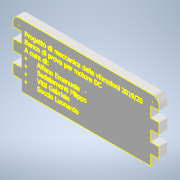
# Autodesk Inventor part: base
Saved by Autodesk Inventor 2020.2 (Build 242310000, 310)
## iProperties
Created: 2020-02-13
Part Number: base
Material: Generico
Document SubType Name: Modeling
Designer: socci
Density: 1 g/cm^3
Appearance: Default
Author: socci
Autodesk Inventor part; units mm, degrees
(part 1 of 5)
ref_plane "YZ Plane" through (0, 0, 0) normal (1, 0, 0) x (0, 1, 0)
ref_plane "XZ Plane" through (0, 0, 0) normal (0, 1, 0) x (-1, 0, 0)
ref_plane "XY Plane" through (0, 0, 0) normal (0, 0, 1) x (1, 0, 0)
sketch "Schizzo1" plane through (0, 0, 0) normal (0, 0, 1) x (1, 0, 0)
  line L0 (-35, -15) -> (35, -15)
  line L1 (35, -15) -> (35, 12)
  line L2 (32, 15) -> (-32, 15)
  line L3 (-35, 12) -> (-35, -15)
  line L4 (-35, -15) -> (35, 15) construction
  line L5 (35, -15) -> (-35, 15) construction
  arc A0 (-32, 15) -> (-35, 12) centre (-32, 12) ccw
  arc A1 (35, 12) -> (32, 15) centre (32, 12) ccw
  point P0 (0, 0)
  dimension "d0" = 70
  dimension "d1" = 30
  dimension "d6" = 3
  constraints: 12 end point, 4 point on circle, 4 point on line, 4 tangent, 2 centre point, 2 midpoint, 2 parallel, 1 equal radius, 1 horizontal, 1 perpendicular
  measures "d0" distance of L4.end L5.end
  measures "d1" distance of L5.end L0.start
  measures "d6" radius of A0
extrude "Estrusione1" add sketch "Schizzo1" along normal blind 4
sketch "Schizzo2" plane through (0, 0, 4) normal (0, 0, 1) x (1, 0, 0)
  line L0 (-29.4007, 10.8975) -> (27.8158, 10.8975) construction
  line L1 (27.8158, 10.8975) -> (27.8158, -22.4613) construction
  line L2 (27.8158, -22.4613) -> (-29.4007, -22.4613) construction
  line L3 (-29.4007, -22.4613) -> (-29.4007, 10.8975) construction
  line L4 (-31, -5) -> (-35, -5)
  line L5 (-35, -5) -> (-35, 0)
  line L6 (-35, 0) -> (-31, 0)
  line L7 (-31, 0) -> (-31, -5)
  line L8 (-35, 10) -> (-31, 10)
  line L9 (-31, 10) -> (-31, 5)
  line L10 (-31, 5) -> (-35, 5)
  line L11 (-35, 5) -> (-35, 10)
  line L12 (-31, -15) -> (-35, -15)
  line L13 (-35, -15) -> (-35, -10)
  line L14 (-35, -10) -> (-31, -10)
  line L15 (-31, -10) -> (-31, -15)
  line L16 (35, -5) -> (31, -5)
  line L17 (31, -5) -> (31, 0)
  line L18 (31, 0) -> (35, 0)
  line L19 (35, 0) -> (35, -5)
  line L20 (31, 10) -> (35, 10)
  line L21 (35, 10) -> (35, 5)
  line L22 (35, 5) -> (31, 5)
  line L23 (31, 5) -> (31, 10)
  line L24 (35, -15) -> (31, -15)
  line L25 (31, -15) -> (31, -10)
  line L26 (31, -10) -> (35, -10)
  line L27 (35, -10) -> (35, -15)
  arc A0 (35, 12) -> (32, 15) centre (32, 12) ccw
  line L28 (35, 12) -> (35, -15)
  line L29 (35, -15) -> (-35, -15)
  line L30 (-35, -15) -> (-35, 12)
  arc A1 (-32, 15) -> (-35, 12) centre (-32, 12) ccw
  line L31 (-32, 15) -> (32, 15)
  spline S0 degree 2 poles (-27.9339, 10.2055) (-27.9339, 10.0758) (-28.0263, 9.8424) (-28.109, 9.7614) knots 0 0 0 1 2 2 2
  spline S1 degree 2 poles (-28.109, 9.7614) (-28.2127, 9.6593) (-28.4931, 9.5539) (-28.707, 9.5539) knots 0 0 0 1 2 2 2
  line L32 (-28.707, 9.5539) -> (-28.9323, 9.5539)
  line L33 (-28.9323, 9.5539) -> (-28.9323, 8.8084)
  line L34 (-28.9323, 8.8084) -> (-29.1981, 8.8084)
  line L35 (-29.1981, 8.8084) -> (-29.1981, 10.8084)
  line L36 (-29.1981, 10.8084) -> (-28.6957, 10.8084)
  spline S2 degree 2 poles (-28.6957, 10.8084) (-28.5174, 10.8084) (-28.2678, 10.75) (-28.1722, 10.6836) knots 0 0 0 1 2 2 2
  spline S3 degree 2 poles (-28.1722, 10.6836) (-28.0603, 10.6074) (-27.9339, 10.3724) (-27.9339, 10.2055) knots 0 0 0 1 2 2 2
  spline S4 degree 2 poles (-28.2111, 10.1974) (-28.2111, 10.3011) (-28.2824, 10.4534) (-28.3553, 10.5021) knots 0 0 0 1 2 2 2
  spline S5 degree 2 poles (-28.3553, 10.5021) (-28.4185, 10.5442) (-28.5871, 10.5782) (-28.7119, 10.5782) knots 0 0 0 1 2 2 2
  line L37 (-28.7119, 10.5782) -> (-28.9323, 10.5782)
  line L38 (-28.9323, 10.5782) -> (-28.9323, 9.7808)
  line L39 (-28.9323, 9.7808) -> (-28.7508, 9.7808)
  spline S6 degree 2 poles (-28.7508, 9.7808) (-28.5887, 9.7808) (-28.3893, 9.8327) (-28.3245, 9.9008) knots 0 0 0 1 2 2 2
  spline S7 degree 2 poles (-28.3245, 9.9008) (-28.2646, 9.9607) (-28.2111, 10.1017) (-28.2111, 10.1974) knots 0 0 0 1 2 2 2
  line L40 (-26.9047, 10.0385) -> (-26.9177, 10.0385)
  spline S8 degree 2 poles (-26.9177, 10.0385) (-26.9469, 10.0466) (-27.0101, 10.0499) (-27.0539, 10.0499) knots 0 0 0 1 2 2 2
  spline S9 degree 2 poles (-27.0539, 10.0499) (-27.156, 10.0499) (-27.3569, 9.9607) (-27.4477, 9.8732) knots 0 0 0 1 2 2 2
  line L41 (-27.4477, 9.8732) -> (-27.4477, 8.8084)
  line L42 (-27.4477, 8.8084) -> (-27.7005, 8.8084)
  line L43 (-27.7005, 8.8084) -> (-27.7005, 10.3092)
  line L44 (-27.7005, 10.3092) -> (-27.4477, 10.3092)
  line L45 (-27.4477, 10.3092) -> (-27.4477, 10.0855)
  spline S10 degree 2 poles (-27.4477, 10.0855) (-27.3099, 10.2087) (-27.1041, 10.3092) (-27.0069, 10.3092) knots 0 0 0 1 2 2 2
  spline S11 degree 2 poles (-27.0069, 10.3092) (-26.968, 10.3092) (-26.9291, 10.306) (-26.9047, 10.3011) knots 0 0 0 1 2 2 2
  line L46 (-26.9047, 10.3011) -> (-26.9047, 10.0385)
  spline S12 degree 2 poles (-25.4752, 9.5588) (-25.4752, 9.1795) (-25.8399, 8.7662) (-26.1446, 8.7662) knots 0 0 0 1 2 2 2
  spline S13 degree 2 poles (-26.1446, 8.7662) (-26.4574, 8.7662) (-26.8156, 9.1925) (-26.8156, 9.5588) knots 0 0 0 1 2 2 2
  spline S14 degree 2 poles (-26.8156, 9.5588) (-26.8156, 9.9348) (-26.4461, 10.3513) (-26.1446, 10.3513) knots 0 0 0 1 2 2 2
  spline S15 degree 2 poles (-26.1446, 10.3513) (-25.8399, 10.3513) (-25.4752, 9.9364) (-25.4752, 9.5588) knots 0 0 0 1 2 2 2
  spline S16 degree 2 poles (-25.7362, 9.5588) (-25.7362, 9.8505) (-25.9485, 10.1342) (-26.1446, 10.1342) knots 0 0 0 1 2 2 2
  spline S17 degree 2 poles (-26.1446, 10.1342) (-26.3407, 10.1342) (-26.5547, 9.8505) (-26.5547, 9.5588) knots 0 0 0 1 2 2 2
  spline S18 degree 2 poles (-26.5547, 9.5588) (-26.5547, 9.2752) (-26.3407, 8.9834) (-26.1446, 8.9834) knots 0 0 0 1 2 2 2
  spline S19 degree 2 poles (-26.1446, 8.9834) (-25.9501, 8.9834) (-25.7362, 9.2703) (-25.7362, 9.5588) knots 0 0 0 1 2 2 2
  spline S20 degree 2 poles (-25.1624, 8.5685) (-25.1365, 8.5572) (-25.0376, 8.5215) (-24.9744, 8.5069) knots 0 0 0 1 2 2 2
  spline S21 degree 2 poles (-24.9744, 8.5069) (-24.9047, 8.4891) (-24.7864, 8.468) (-24.7167, 8.468) knots 0 0 0 1 2 2 2
  spline S22 degree 2 poles (-24.7167, 8.468) (-24.6, 8.468) (-24.438, 8.5296) (-24.3926, 8.5847) knots 0 0 0 1 2 2 2
  spline S23 degree 2 poles (-24.3926, 8.5847) (-24.3488, 8.6398) (-24.3148, 8.7841) (-24.3148, 8.8765) knots 0 0 0 1 2 2 2
  line L47 (-24.3148, 8.8765) -> (-24.3148, 9.0077)
  spline S24 degree 2 poles (-24.3148, 9.0077) (-24.4169, 8.9186) (-24.613, 8.8343) (-24.7605, 8.8343) knots 0 0 0 1 2 2 2
  spline S25 degree 2 poles (-24.7605, 8.8343) (-25.0166, 8.8343) (-25.3197, 9.2152) (-25.3197, 9.5734) knots 0 0 0 1 2 2 2
  spline S26 degree 2 poles (-25.3197, 9.5734) (-25.3197, 9.7598) (-25.2143, 10.0483) (-25.1268, 10.1504) knots 0 0 0 1 2 2 2
  spline S27 degree 2 poles (-25.1268, 10.1504) (-25.0425, 10.246) (-24.8107, 10.3513) (-24.6876, 10.3513) knots 0 0 0 1 2 2 2
  spline S28 degree 2 poles (-24.6876, 10.3513) (-24.5709, 10.3513) (-24.4007, 10.2962) (-24.3148, 10.246) knots 0 0 0 1 2 2 2
  line L48 (-24.3148, 10.246) -> (-24.3002, 10.3092)
  line L49 (-24.3002, 10.3092) -> (-24.062, 10.3092)
  line L50 (-24.062, 10.3092) -> (-24.062, 8.9802)
  spline S29 degree 2 poles (-24.062, 8.9802) (-24.062, 8.5977) (-24.3942, 8.2411) (-24.7362, 8.2411) knots 0 0 0 1 2 2 2
  spline S30 degree 2 poles (-24.7362, 8.2411) (-24.8464, 8.2411) (-25.0765, 8.2768) (-25.1754, 8.306) knots 0 0 0 1 2 2 2
  line L51 (-25.1754, 8.306) -> (-25.1754, 8.5685)
  line L52 (-25.1754, 8.5685) -> (-25.1624, 8.5685)
  line L53 (-24.3148, 9.2152) -> (-24.3148, 10.0402)
  spline S31 degree 2 poles (-24.3148, 10.0402) (-24.4088, 10.0855) (-24.5676, 10.1244) (-24.647, 10.1244) knots 0 0 0 1 2 2 2
  spline S32 degree 2 poles (-24.647, 10.1244) (-24.8383, 10.1244) (-25.0587, 9.8424) (-25.0587, 9.5782) knots 0 0 0 1 2 2 2
  spline S33 degree 2 poles (-25.0587, 9.5782) (-25.0587, 9.3286) (-24.8918, 9.0677) (-24.7038, 9.0677) knots 0 0 0 1 2 2 2
  spline S34 degree 2 poles (-24.7038, 9.0677) (-24.6049, 9.0677) (-24.3975, 9.1455) (-24.3148, 9.2152) knots 0 0 0 1 2 2 2
  spline S35 degree 2 poles (-23.0441, 8.7743) (-23.4039, 8.7743) (-23.7994, 9.1779) (-23.7994, 9.5507) knots 0 0 0 1 2 2 2
  spline S36 degree 2 poles (-23.7994, 9.5507) (-23.7994, 9.917) (-23.4153, 10.3513) (-23.1057, 10.3513) knots 0 0 0 1 2 2 2
  spline S37 degree 2 poles (-23.1057, 10.3513) (-22.9663, 10.3513) (-22.7508, 10.2703) (-22.6714, 10.1844) knots 0 0 0 1 2 2 2
  spline S38 degree 2 poles (-22.6714, 10.1844) (-22.5903, 10.0985) (-22.5044, 9.8505) (-22.5044, 9.6706) knots 0 0 0 1 2 2 2
  line L54 (-22.5044, 9.6706) -> (-22.5044, 9.5329)
  line L55 (-22.5044, 9.5329) -> (-23.5433, 9.5329)
  spline S39 degree 2 poles (-23.5433, 9.5329) (-23.5433, 9.2719) (-23.2808, 8.9948) (-23.0474, 8.9948) knots 0 0 0 1 2 2 2
  spline S40 degree 2 poles (-23.0474, 8.9948) (-22.9647, 8.9948) (-22.8043, 9.032) (-22.7394, 9.0612) knots 0 0 0 1 2 2 2
  spline S41 degree 2 poles (-22.7394, 9.0612) (-22.6714, 9.0936) (-22.5774, 9.1504) (-22.5466, 9.1763) knots 0 0 0 1 2 2 2
  line L56 (-22.5466, 9.1763) -> (-22.532, 9.1763)
  line L57 (-22.532, 9.1763) -> (-22.532, 8.9008)
  spline S42 degree 2 poles (-22.532, 8.9008) (-22.5757, 8.8829) (-22.7086, 8.8311) (-22.7605, 8.8165) knots 0 0 0 1 2 2 2
  spline S43 degree 2 poles (-22.7605, 8.8165) (-22.8334, 8.7954) (-22.9534, 8.7743) (-23.0441, 8.7743) knots 0 0 0 1 2 2 2
  spline S44 degree 2 poles (-22.7508, 9.7257) (-22.754, 9.8278) (-22.7962, 9.9769) (-22.8367, 10.0272) knots 0 0 0 1 2 2 2
  spline S45 degree 2 poles (-22.8367, 10.0272) (-22.8804, 10.0839) (-23.0182, 10.1439) (-23.1203, 10.1439) knots 0 0 0 1 2 2 2
  spline S46 degree 2 poles (-23.1203, 10.1439) (-23.2208, 10.1439) (-23.3618, 10.0839) (-23.4201, 10.0256) knots 0 0 0 1 2 2 2
  spline S47 degree 2 poles (-23.4201, 10.0256) (-23.4769, 9.9656) (-23.5352, 9.8214) (-23.5433, 9.7257) knots 0 0 0 1 2 2 2
  line L58 (-23.5433, 9.7257) -> (-22.7508, 9.7257)
  spline S48 degree 2 poles (-21.7945, 8.7792) (-22.0004, 8.7792) (-22.2321, 9.0142) (-22.2321, 9.2687) knots 0 0 0 1 2 2 2
  line L59 (-22.2321, 9.2687) -> (-22.2321, 10.1001)
  line L60 (-22.2321, 10.1001) -> (-22.4023, 10.1001)
  line L61 (-22.4023, 10.1001) -> (-22.4023, 10.3092)
  line L62 (-22.4023, 10.3092) -> (-22.2321, 10.3092)
  line L63 (-22.2321, 10.3092) -> (-22.2321, 10.7403)
  line L64 (-22.2321, 10.7403) -> (-21.9793, 10.7403)
  line L65 (-21.9793, 10.7403) -> (-21.9793, 10.3092)
  line L66 (-21.9793, 10.3092) -> (-21.5141, 10.3092)
  line L67 (-21.5141, 10.3092) -> (-21.5141, 10.1001)
  line L68 (-21.5141, 10.1001) -> (-21.9793, 10.1001)
  line L69 (-21.9793, 10.1001) -> (-21.9793, 9.3854)
  spline S49 degree 2 poles (-21.9793, 9.3854) (-21.9793, 9.2719) (-21.9712, 9.1471) (-21.9436, 9.0936) knots 0 0 0 1 2 2 2
  spline S50 degree 2 poles (-21.9436, 9.0936) (-21.921, 9.0466) (-21.8188, 8.9996) (-21.7313, 8.9996) knots 0 0 0 1 2 2 2
  spline S51 degree 2 poles (-21.7313, 8.9996) (-21.6697, 8.9996) (-21.5547, 9.0369) (-21.5287, 9.0483) knots 0 0 0 1 2 2 2
  line L70 (-21.5287, 9.0483) -> (-21.5141, 9.0483)
  line L71 (-21.5141, 9.0483) -> (-21.5141, 8.8214)
  spline S52 degree 2 poles (-21.5141, 8.8214) (-21.5855, 8.8019) (-21.7313, 8.7792) (-21.7945, 8.7792) knots 0 0 0 1 2 2 2
  spline S53 degree 2 poles (-20.874, 8.7792) (-21.0798, 8.7792) (-21.3116, 9.0142) (-21.3116, 9.2687) knots 0 0 0 1 2 2 2
  line L72 (-21.3116, 9.2687) -> (-21.3116, 10.1001)
  line L73 (-21.3116, 10.1001) -> (-21.4817, 10.1001)
  line L74 (-21.4817, 10.1001) -> (-21.4817, 10.3092)
  line L75 (-21.4817, 10.3092) -> (-21.3116, 10.3092)
  line L76 (-21.3116, 10.3092) -> (-21.3116, 10.7403)
  line L77 (-21.3116, 10.7403) -> (-21.0587, 10.7403)
  line L78 (-21.0587, 10.7403) -> (-21.0587, 10.3092)
  line L79 (-21.0587, 10.3092) -> (-20.5936, 10.3092)
  line L80 (-20.5936, 10.3092) -> (-20.5936, 10.1001)
  line L81 (-20.5936, 10.1001) -> (-21.0587, 10.1001)
  line L82 (-21.0587, 10.1001) -> (-21.0587, 9.3854)
  spline S54 degree 2 poles (-21.0587, 9.3854) (-21.0587, 9.2719) (-21.0506, 9.1471) (-21.0231, 9.0936) knots 0 0 0 1 2 2 2
  spline S55 degree 2 poles (-21.0231, 9.0936) (-21.0004, 9.0466) (-20.8983, 8.9996) (-20.8107, 8.9996) knots 0 0 0 1 2 2 2
  spline S56 degree 2 poles (-20.8107, 8.9996) (-20.7492, 8.9996) (-20.6341, 9.0369) (-20.6081, 9.0483) knots 0 0 0 1 2 2 2
  line L83 (-20.6081, 9.0483) -> (-20.5936, 9.0483)
  line L84 (-20.5936, 9.0483) -> (-20.5936, 8.8214)
  spline S57 degree 2 poles (-20.5936, 8.8214) (-20.6649, 8.8019) (-20.8107, 8.7792) (-20.874, 8.7792) knots 0 0 0 1 2 2 2
  spline S58 degree 2 poles (-19.1738, 9.5588) (-19.1738, 9.1795) (-19.5385, 8.7662) (-19.8432, 8.7662) knots 0 0 0 1 2 2 2
  spline S59 degree 2 poles (-19.8432, 8.7662) (-20.156, 8.7662) (-20.5141, 9.1925) (-20.5141, 9.5588) knots 0 0 0 1 2 2 2
  spline S60 degree 2 poles (-20.5141, 9.5588) (-20.5141, 9.9348) (-20.1446, 10.3513) (-19.8432, 10.3513) knots 0 0 0 1 2 2 2
  spline S61 degree 2 poles (-19.8432, 10.3513) (-19.5385, 10.3513) (-19.1738, 9.9364) (-19.1738, 9.5588) knots 0 0 0 1 2 2 2
  spline S62 degree 2 poles (-19.4347, 9.5588) (-19.4347, 9.8505) (-19.647, 10.1342) (-19.8432, 10.1342) knots 0 0 0 1 2 2 2
  spline S63 degree 2 poles (-19.8432, 10.1342) (-20.0393, 10.1342) (-20.2532, 9.8505) (-20.2532, 9.5588) knots 0 0 0 1 2 2 2
  spline S64 degree 2 poles (-20.2532, 9.5588) (-20.2532, 9.2752) (-20.0393, 8.9834) (-19.8432, 8.9834) knots 0 0 0 1 2 2 2
  spline S65 degree 2 poles (-19.8432, 8.9834) (-19.6487, 8.9834) (-19.4347, 9.2703) (-19.4347, 9.5588) knots 0 0 0 1 2 2 2
  line L85 (-16.9015, 8.8084) -> (-17.1543, 8.8084)
  line L86 (-17.1543, 8.8084) -> (-17.1543, 8.9607)
  spline S66 degree 2 poles (-17.1543, 8.9607) (-17.2127, 8.9121) (-17.2986, 8.8473) (-17.3569, 8.8197) knots 0 0 0 1 2 2 2
  spline S67 degree 2 poles (-17.3569, 8.8197) (-17.4104, 8.7938) (-17.5255, 8.7662) (-17.6017, 8.7662) knots 0 0 0 1 2 2 2
  spline S68 degree 2 poles (-17.6017, 8.7662) (-17.7248, 8.7662) (-17.9323, 8.8684) (-18.0052, 8.9672) knots 0 0 0 1 2 2 2
  spline S69 degree 2 poles (-18.0052, 8.9672) (-18.0782, 9.0661) (-18.1592, 9.3578) (-18.1592, 9.5474) knots 0 0 0 1 2 2 2
  spline S70 degree 2 poles (-18.1592, 9.5474) (-18.1592, 9.7452) (-18.0571, 10.0337) (-17.968, 10.1423) knots 0 0 0 1 2 2 2
  spline S71 degree 2 poles (-17.968, 10.1423) (-17.8853, 10.2395) (-17.6535, 10.3513) (-17.5255, 10.3513) knots 0 0 0 1 2 2 2
  spline S72 degree 2 poles (-17.5255, 10.3513) (-17.4137, 10.3513) (-17.2467, 10.3011) (-17.1543, 10.2492) knots 0 0 0 1 2 2 2
  line L87 (-17.1543, 10.2492) -> (-17.1543, 10.8975)
  line L88 (-17.1543, 10.8975) -> (-16.9015, 10.8975)
  line L89 (-16.9015, 10.8975) -> (-16.9015, 8.8084)
  line L90 (-17.1543, 9.1731) -> (-17.1543, 10.0402)
  spline S73 degree 2 poles (-17.1543, 10.0402) (-17.2483, 10.0855) (-17.3975, 10.1196) (-17.4834, 10.1196) knots 0 0 0 1 2 2 2
  spline S74 degree 2 poles (-17.4834, 10.1196) (-17.6778, 10.1196) (-17.8983, 9.8278) (-17.8983, 9.5523) knots 0 0 0 1 2 2 2
  spline S75 degree 2 poles (-17.8983, 9.5523) (-17.8983, 9.2865) (-17.7297, 9.0061) (-17.5433, 9.0061) knots 0 0 0 1 2 2 2
  spline S76 degree 2 poles (-17.5433, 9.0061) (-17.4445, 9.0061) (-17.2435, 9.0969) (-17.1543, 9.1731) knots 0 0 0 1 2 2 2
  line L91 (-16.2775, 8.8084) -> (-16.5304, 8.8084)
  line L92 (-16.5304, 8.8084) -> (-16.5304, 10.3092)
  line L93 (-16.5304, 10.3092) -> (-16.2775, 10.3092)
  line L94 (-16.2775, 10.3092) -> (-16.2775, 8.8084)
  line L95 (-16.2597, 10.5588) -> (-16.5466, 10.5588)
  line L96 (-16.5466, 10.5588) -> (-16.5466, 10.8214)
  line L97 (-16.5466, 10.8214) -> (-16.2597, 10.8214)
  line L98 (-16.2597, 10.8214) -> (-16.2597, 10.5588)
  line L99 (-13.3456, 8.8084) -> (-13.3456, 9.6771)
  spline S77 degree 2 poles (-13.3456, 9.6771) (-13.3456, 9.7808) (-13.3618, 9.9575) (-13.3877, 10.0061) knots 0 0 0 1 2 2 2
  spline S78 degree 2 poles (-13.3877, 10.0061) (-13.4137, 10.0596) (-13.5125, 10.1115) (-13.5984, 10.1115) knots 0 0 0 1 2 2 2
  spline S79 degree 2 poles (-13.5984, 10.1115) (-13.6762, 10.1115) (-13.8545, 10.0158) (-13.9485, 9.9251) knots 0 0 0 1 2 2 2
  spline S80 degree 2 poles (-13.9485, 9.9251) (-13.9469, 9.9024) (-13.9436, 9.8392) (-13.9436, 9.797) knots 0 0 0 1 2 2 2
  line L100 (-13.9436, 9.797) -> (-13.9436, 8.8084)
  line L101 (-13.9436, 8.8084) -> (-14.1965, 8.8084)
  line L102 (-14.1965, 8.8084) -> (-14.1965, 9.6771)
  spline S81 degree 2 poles (-14.1965, 9.6771) (-14.1965, 9.7808) (-14.2127, 9.9575) (-14.2386, 10.0061) knots 0 0 0 1 2 2 2
  spline S82 degree 2 poles (-14.2386, 10.0061) (-14.2646, 10.0596) (-14.3634, 10.1115) (-14.4493, 10.1115) knots 0 0 0 1 2 2 2
  spline S83 degree 2 poles (-14.4493, 10.1115) (-14.5304, 10.1115) (-14.7103, 10.0094) (-14.7945, 9.9299) knots 0 0 0 1 2 2 2
  line L103 (-14.7945, 9.9299) -> (-14.7945, 8.8084)
  line L104 (-14.7945, 8.8084) -> (-15.0474, 8.8084)
  line L105 (-15.0474, 8.8084) -> (-15.0474, 10.3092)
  line L106 (-15.0474, 10.3092) -> (-14.7945, 10.3092)
  line L107 (-14.7945, 10.3092) -> (-14.7945, 10.1439)
  spline S84 degree 2 poles (-14.7945, 10.1439) (-14.6957, 10.2427) (-14.5012, 10.3513) (-14.3845, 10.3513) knots 0 0 0 1 2 2 2
  spline S85 degree 2 poles (-14.3845, 10.3513) (-14.2516, 10.3513) (-14.0458, 10.2298) (-13.9923, 10.092) knots 0 0 0 1 2 2 2
  spline S86 degree 2 poles (-13.9923, 10.092) (-13.8772, 10.2201) (-13.66, 10.3513) (-13.5336, 10.3513) knots 0 0 0 1 2 2 2
  spline S87 degree 2 poles (-13.5336, 10.3513) (-13.4364, 10.3513) (-13.2775, 10.2914) (-13.2192, 10.2233) knots 0 0 0 1 2 2 2
  spline S88 degree 2 poles (-13.2192, 10.2233) (-13.1592, 10.1552) (-13.0928, 9.951) (-13.0928, 9.797) knots 0 0 0 1 2 2 2
  line L108 (-13.0928, 9.797) -> (-13.0928, 8.8084)
  line L109 (-13.0928, 8.8084) -> (-13.3456, 8.8084)
  spline S89 degree 2 poles (-12.0863, 8.7743) (-12.4461, 8.7743) (-12.8415, 9.1779) (-12.8415, 9.5507) knots 0 0 0 1 2 2 2
  spline S90 degree 2 poles (-12.8415, 9.5507) (-12.8415, 9.917) (-12.4574, 10.3513) (-12.1479, 10.3513) knots 0 0 0 1 2 2 2
  spline S91 degree 2 poles (-12.1479, 10.3513) (-12.0085, 10.3513) (-11.7929, 10.2703) (-11.7135, 10.1844) knots 0 0 0 1 2 2 2
  spline S92 degree 2 poles (-11.7135, 10.1844) (-11.6325, 10.0985) (-11.5466, 9.8505) (-11.5466, 9.6706) knots 0 0 0 1 2 2 2
  line L110 (-11.5466, 9.6706) -> (-11.5466, 9.5329)
  line L111 (-11.5466, 9.5329) -> (-12.5855, 9.5329)
  spline S93 degree 2 poles (-12.5855, 9.5329) (-12.5855, 9.2719) (-12.3229, 8.9948) (-12.0895, 8.9948) knots 0 0 0 1 2 2 2
  spline S94 degree 2 poles (-12.0895, 8.9948) (-12.0069, 8.9948) (-11.8464, 9.032) (-11.7816, 9.0612) knots 0 0 0 1 2 2 2
  spline S95 degree 2 poles (-11.7816, 9.0612) (-11.7135, 9.0936) (-11.6195, 9.1504) (-11.5887, 9.1763) knots 0 0 0 1 2 2 2
  line L112 (-11.5887, 9.1763) -> (-11.5741, 9.1763)
  line L113 (-11.5741, 9.1763) -> (-11.5741, 8.9008)
  spline S96 degree 2 poles (-11.5741, 8.9008) (-11.6179, 8.8829) (-11.7508, 8.8311) (-11.8026, 8.8165) knots 0 0 0 1 2 2 2
  spline S97 degree 2 poles (-11.8026, 8.8165) (-11.8756, 8.7954) (-11.9955, 8.7743) (-12.0863, 8.7743) knots 0 0 0 1 2 2 2
  spline S98 degree 2 poles (-11.7929, 9.7257) (-11.7962, 9.8278) (-11.8383, 9.9769) (-11.8788, 10.0272) knots 0 0 0 1 2 2 2
  spline S99 degree 2 poles (-11.8788, 10.0272) (-11.9226, 10.0839) (-12.0603, 10.1439) (-12.1624, 10.1439) knots 0 0 0 1 2 2 2
  spline S100 degree 2 poles (-12.1624, 10.1439) (-12.2629, 10.1439) (-12.4039, 10.0839) (-12.4623, 10.0256) knots 0 0 0 1 2 2 2
  spline S101 degree 2 poles (-12.4623, 10.0256) (-12.519, 9.9656) (-12.5774, 9.8214) (-12.5855, 9.7257) knots 0 0 0 1 2 2 2
  line L114 (-12.5855, 9.7257) -> (-11.7929, 9.7257)
  spline S102 degree 2 poles (-10.694, 8.7743) (-10.8496, 8.7743) (-11.1073, 8.87) (-11.1997, 8.9672) knots 0 0 0 1 2 2 2
  spline S103 degree 2 poles (-11.1997, 8.9672) (-11.2921, 9.0628) (-11.3942, 9.3578) (-11.3942, 9.5555) knots 0 0 0 1 2 2 2
  spline S104 degree 2 poles (-11.3942, 9.5555) (-11.3942, 9.7533) (-11.2889, 10.0418) (-11.1997, 10.139) knots 0 0 0 1 2 2 2
  spline S105 degree 2 poles (-11.1997, 10.139) (-11.1106, 10.2379) (-10.8464, 10.3432) (-10.694, 10.3432) knots 0 0 0 1 2 2 2
  spline S106 degree 2 poles (-10.694, 10.3432) (-10.5709, 10.3432) (-10.3407, 10.2735) (-10.2516, 10.2282) knots 0 0 0 1 2 2 2
  line L115 (-10.2516, 10.2282) -> (-10.2516, 9.9445)
  line L116 (-10.2516, 9.9445) -> (-10.2662, 9.9445)
  spline S107 degree 2 poles (-10.2662, 9.9445) (-10.2937, 9.9672) (-10.378, 10.0256) (-10.438, 10.0564) knots 0 0 0 1 2 2 2
  spline S108 degree 2 poles (-10.438, 10.0564) (-10.4915, 10.0823) (-10.6341, 10.1228) (-10.6989, 10.1228) knots 0 0 0 1 2 2 2
  spline S109 degree 2 poles (-10.6989, 10.1228) (-10.895, 10.1228) (-11.1333, 9.8262) (-11.1333, 9.5555) knots 0 0 0 1 2 2 2
  spline S110 degree 2 poles (-11.1333, 9.5555) (-11.1333, 9.2914) (-10.9031, 8.9948) (-10.6989, 8.9948) knots 0 0 0 1 2 2 2
  spline S111 degree 2 poles (-10.6989, 8.9948) (-10.5757, 8.9948) (-10.3521, 9.0969) (-10.2662, 9.1763) knots 0 0 0 1 2 2 2
  line L117 (-10.2662, 9.1763) -> (-10.2516, 9.1763)
  line L118 (-10.2516, 9.1763) -> (-10.2516, 8.8927)
  spline S112 degree 2 poles (-10.2516, 8.8927) (-10.2889, 8.8748) (-10.4023, 8.8246) (-10.4477, 8.8132) knots 0 0 0 1 2 2 2
  spline S113 degree 2 poles (-10.4477, 8.8132) (-10.5125, 8.7938) (-10.6146, 8.7743) (-10.694, 8.7743) knots 0 0 0 1 2 2 2
  spline S114 degree 2 poles (-9.425, 8.7743) (-9.5806, 8.7743) (-9.8383, 8.87) (-9.9307, 8.9672) knots 0 0 0 1 2 2 2
  spline S115 degree 2 poles (-9.9307, 8.9672) (-10.0231, 9.0628) (-10.1252, 9.3578) (-10.1252, 9.5555) knots 0 0 0 1 2 2 2
  spline S116 degree 2 poles (-10.1252, 9.5555) (-10.1252, 9.7533) (-10.0198, 10.0418) (-9.9307, 10.139) knots 0 0 0 1 2 2 2
  spline S117 degree 2 poles (-9.9307, 10.139) (-9.8415, 10.2379) (-9.5774, 10.3432) (-9.425, 10.3432) knots 0 0 0 1 2 2 2
  spline S118 degree 2 poles (-9.425, 10.3432) (-9.3018, 10.3432) (-9.0717, 10.2735) (-8.9825, 10.2282) knots 0 0 0 1 2 2 2
  line L119 (-8.9825, 10.2282) -> (-8.9825, 9.9445)
  line L120 (-8.9825, 9.9445) -> (-8.9971, 9.9445)
  spline S119 degree 2 poles (-8.9971, 9.9445) (-9.0247, 9.9672) (-9.109, 10.0256) (-9.1689, 10.0564) knots 0 0 0 1 2 2 2
  spline S120 degree 2 poles (-9.1689, 10.0564) (-9.2224, 10.0823) (-9.365, 10.1228) (-9.4299, 10.1228) knots 0 0 0 1 2 2 2
  spline S121 degree 2 poles (-9.4299, 10.1228) (-9.626, 10.1228) (-9.8642, 9.8262) (-9.8642, 9.5555) knots 0 0 0 1 2 2 2
  spline S122 degree 2 poles (-9.8642, 9.5555) (-9.8642, 9.2914) (-9.6341, 8.9948) (-9.4299, 8.9948) knots 0 0 0 1 2 2 2
  spline S123 degree 2 poles (-9.4299, 8.9948) (-9.3067, 8.9948) (-9.083, 9.0969) (-8.9971, 9.1763) knots 0 0 0 1 2 2 2
  line L121 (-8.9971, 9.1763) -> (-8.9825, 9.1763)
  line L122 (-8.9825, 9.1763) -> (-8.9825, 8.8927)
  spline S124 degree 2 poles (-8.9825, 8.8927) (-9.0198, 8.8748) (-9.1333, 8.8246) (-9.1787, 8.8132) knots 0 0 0 1 2 2 2
  spline S125 degree 2 poles (-9.1787, 8.8132) (-9.2435, 8.7938) (-9.3456, 8.7743) (-9.425, 8.7743) knots 0 0 0 1 2 2 2
  spline S126 degree 2 poles (-7.9161, 8.9672) (-7.9469, 8.9445) (-8.0506, 8.8635) (-8.0992, 8.8392) knots 0 0 0 1 2 2 2
  spline S127 degree 2 poles (-8.0992, 8.8392) (-8.1657, 8.8035) (-8.2905, 8.7662) (-8.4039, 8.7662) knots 0 0 0 1 2 2 2
  spline S128 degree 2 poles (-8.4039, 8.7662) (-8.4963, 8.7662) (-8.6633, 8.8359) (-8.7265, 8.8991) knots 0 0 0 1 2 2 2
  spline S129 degree 2 poles (-8.7265, 8.8991) (-8.7864, 8.9607) (-8.8594, 9.1423) (-8.8594, 9.2427) knots 0 0 0 1 2 2 2
  spline S130 degree 2 poles (-8.8594, 9.2427) (-8.8594, 9.3983) (-8.7281, 9.6188) (-8.5855, 9.682) knots 0 0 0 1 2 2 2
  spline S131 degree 2 poles (-8.5855, 9.682) (-8.459, 9.7403) (-8.1154, 9.7841) (-7.9161, 9.7954) knots 0 0 0 1 2 2 2
  line L123 (-7.9161, 9.7954) -> (-7.9161, 9.844)
  spline S132 degree 2 poles (-7.9161, 9.844) (-7.9161, 9.9316) (-7.9696, 10.0402) (-8.0182, 10.0709) knots 0 0 0 1 2 2 2
  spline S133 degree 2 poles (-8.0182, 10.0709) (-8.0668, 10.1017) (-8.2062, 10.1212) (-8.2808, 10.1212) knots 0 0 0 1 2 2 2
  spline S134 degree 2 poles (-8.2808, 10.1212) (-8.3683, 10.1212) (-8.6049, 10.0693) (-8.7232, 10.0191) knots 0 0 0 1 2 2 2
  line L124 (-8.7232, 10.0191) -> (-8.7378, 10.0191)
  line L125 (-8.7378, 10.0191) -> (-8.7378, 10.2768)
  spline S135 degree 2 poles (-8.7378, 10.2768) (-8.6681, 10.2962) (-8.4072, 10.3449) (-8.2791, 10.3449) knots 0 0 0 1 2 2 2
  spline S136 degree 2 poles (-8.2791, 10.3449) (-8.1235, 10.3449) (-7.9112, 10.2962) (-7.8269, 10.233) knots 0 0 0 1 2 2 2
  spline S137 degree 2 poles (-7.8269, 10.233) (-7.7443, 10.1714) (-7.6633, 9.9753) (-7.6633, 9.8343) knots 0 0 0 1 2 2 2
  line L126 (-7.6633, 9.8343) -> (-7.6633, 8.8084)
  line L127 (-7.6633, 8.8084) -> (-7.9161, 8.8084)
  line L128 (-7.9161, 8.8084) -> (-7.9161, 8.9672)
  line L129 (-7.9161, 9.1779) -> (-7.9161, 9.5944)
  spline S138 degree 2 poles (-7.9161, 9.5944) (-8.0069, 9.5863) (-8.2808, 9.5588) (-8.3667, 9.5329) knots 0 0 0 1 2 2 2
  spline S139 degree 2 poles (-8.3667, 9.5329) (-8.4671, 9.5021) (-8.5984, 9.374) (-8.5984, 9.2606) knots 0 0 0 1 2 2 2
  spline S140 degree 2 poles (-8.5984, 9.2606) (-8.5984, 9.1309) (-8.4526, 8.9996) (-8.3132, 8.9996) knots 0 0 0 1 2 2 2
  spline S141 degree 2 poles (-8.3132, 8.9996) (-8.1949, 8.9996) (-8.0004, 9.1017) (-7.9161, 9.1779) knots 0 0 0 1 2 2 2
  line L130 (-6.13, 8.8084) -> (-6.3829, 8.8084)
  line L131 (-6.3829, 8.8084) -> (-6.3829, 9.6641)
  spline S142 degree 2 poles (-6.3829, 9.6641) (-6.3829, 9.7679) (-6.4023, 9.9461) (-6.4315, 9.9996) knots 0 0 0 1 2 2 2
  spline S143 degree 2 poles (-6.4315, 9.9996) (-6.4623, 10.0564) (-6.5725, 10.1115) (-6.6665, 10.1115) knots 0 0 0 1 2 2 2
  spline S144 degree 2 poles (-6.6665, 10.1115) (-6.7605, 10.1115) (-6.9599, 10.011) (-7.0555, 9.9299) knots 0 0 0 1 2 2 2
  line L132 (-7.0555, 9.9299) -> (-7.0555, 8.8084)
  line L133 (-7.0555, 8.8084) -> (-7.3083, 8.8084)
  line L134 (-7.3083, 8.8084) -> (-7.3083, 10.3092)
  line L135 (-7.3083, 10.3092) -> (-7.0555, 10.3092)
  line L136 (-7.0555, 10.3092) -> (-7.0555, 10.1423)
  spline S145 degree 2 poles (-7.0555, 10.1423) (-6.942, 10.2444) (-6.7232, 10.3513) (-6.6, 10.3513) knots 0 0 0 1 2 2 2
  spline S146 degree 2 poles (-6.6, 10.3513) (-6.3796, 10.3513) (-6.13, 10.0596) (-6.13, 9.7825) knots 0 0 0 1 2 2 2
  line L137 (-6.13, 9.7825) -> (-6.13, 8.8084)
  line L138 (-5.5174, 8.8084) -> (-5.7702, 8.8084)
  line L139 (-5.7702, 8.8084) -> (-5.7702, 10.3092)
  line L140 (-5.7702, 10.3092) -> (-5.5174, 10.3092)
  line L141 (-5.5174, 10.3092) -> (-5.5174, 8.8084)
  line L142 (-5.4996, 10.5588) -> (-5.7864, 10.5588)
  line L143 (-5.7864, 10.5588) -> (-5.7864, 10.8214)
  line L144 (-5.7864, 10.8214) -> (-5.4996, 10.8214)
  line L145 (-5.4996, 10.8214) -> (-5.4996, 10.5588)
  spline S147 degree 2 poles (-4.5498, 8.7743) (-4.7054, 8.7743) (-4.9631, 8.87) (-5.0555, 8.9672) knots 0 0 0 1 2 2 2
  spline S148 degree 2 poles (-5.0555, 8.9672) (-5.1479, 9.0628) (-5.25, 9.3578) (-5.25, 9.5555) knots 0 0 0 1 2 2 2
  spline S149 degree 2 poles (-5.25, 9.5555) (-5.25, 9.7533) (-5.1446, 10.0418) (-5.0555, 10.139) knots 0 0 0 1 2 2 2
  spline S150 degree 2 poles (-5.0555, 10.139) (-4.9663, 10.2379) (-4.7022, 10.3432) (-4.5498, 10.3432) knots 0 0 0 1 2 2 2
  spline S151 degree 2 poles (-4.5498, 10.3432) (-4.4266, 10.3432) (-4.1965, 10.2735) (-4.1073, 10.2282) knots 0 0 0 1 2 2 2
  line L146 (-4.1073, 10.2282) -> (-4.1073, 9.9445)
  line L147 (-4.1073, 9.9445) -> (-4.1219, 9.9445)
  spline S152 degree 2 poles (-4.1219, 9.9445) (-4.1495, 9.9672) (-4.2338, 10.0256) (-4.2937, 10.0564) knots 0 0 0 1 2 2 2
  spline S153 degree 2 poles (-4.2937, 10.0564) (-4.3472, 10.0823) (-4.4898, 10.1228) (-4.5547, 10.1228) knots 0 0 0 1 2 2 2
  spline S154 degree 2 poles (-4.5547, 10.1228) (-4.7508, 10.1228) (-4.989, 9.8262) (-4.989, 9.5555) knots 0 0 0 1 2 2 2
  spline S155 degree 2 poles (-4.989, 9.5555) (-4.989, 9.2914) (-4.7589, 8.9948) (-4.5547, 8.9948) knots 0 0 0 1 2 2 2
  spline S156 degree 2 poles (-4.5547, 8.9948) (-4.4315, 8.9948) (-4.2078, 9.0969) (-4.1219, 9.1763) knots 0 0 0 1 2 2 2
  line L148 (-4.1219, 9.1763) -> (-4.1073, 9.1763)
  line L149 (-4.1073, 9.1763) -> (-4.1073, 8.8927)
  spline S157 degree 2 poles (-4.1073, 8.8927) (-4.1446, 8.8748) (-4.2581, 8.8246) (-4.3034, 8.8132) knots 0 0 0 1 2 2 2
  spline S158 degree 2 poles (-4.3034, 8.8132) (-4.3683, 8.7938) (-4.4704, 8.7743) (-4.5498, 8.7743) knots 0 0 0 1 2 2 2
  spline S159 degree 2 poles (-3.0409, 8.9672) (-3.0717, 8.9445) (-3.1754, 8.8635) (-3.224, 8.8392) knots 0 0 0 1 2 2 2
  spline S160 degree 2 poles (-3.224, 8.8392) (-3.2905, 8.8035) (-3.4153, 8.7662) (-3.5287, 8.7662) knots 0 0 0 1 2 2 2
  spline S161 degree 2 poles (-3.5287, 8.7662) (-3.6211, 8.7662) (-3.7881, 8.8359) (-3.8513, 8.8991) knots 0 0 0 1 2 2 2
  spline S162 degree 2 poles (-3.8513, 8.8991) (-3.9112, 8.9607) (-3.9842, 9.1423) (-3.9842, 9.2427) knots 0 0 0 1 2 2 2
  spline S163 degree 2 poles (-3.9842, 9.2427) (-3.9842, 9.3983) (-3.8529, 9.6188) (-3.7103, 9.682) knots 0 0 0 1 2 2 2
  spline S164 degree 2 poles (-3.7103, 9.682) (-3.5838, 9.7403) (-3.2402, 9.7841) (-3.0409, 9.7954) knots 0 0 0 1 2 2 2
  line L150 (-3.0409, 9.7954) -> (-3.0409, 9.844)
  spline S165 degree 2 poles (-3.0409, 9.844) (-3.0409, 9.9316) (-3.0944, 10.0402) (-3.143, 10.0709) knots 0 0 0 1 2 2 2
  spline S166 degree 2 poles (-3.143, 10.0709) (-3.1916, 10.1017) (-3.331, 10.1212) (-3.4056, 10.1212) knots 0 0 0 1 2 2 2
  spline S167 degree 2 poles (-3.4056, 10.1212) (-3.4931, 10.1212) (-3.7297, 10.0693) (-3.848, 10.0191) knots 0 0 0 1 2 2 2
  line L151 (-3.848, 10.0191) -> (-3.8626, 10.0191)
  line L152 (-3.8626, 10.0191) -> (-3.8626, 10.2768)
  spline S168 degree 2 poles (-3.8626, 10.2768) (-3.7929, 10.2962) (-3.532, 10.3449) (-3.4039, 10.3449) knots 0 0 0 1 2 2 2
  spline S169 degree 2 poles (-3.4039, 10.3449) (-3.2483, 10.3449) (-3.036, 10.2962) (-2.9517, 10.233) knots 0 0 0 1 2 2 2
  spline S170 degree 2 poles (-2.9517, 10.233) (-2.8691, 10.1714) (-2.7881, 9.9753) (-2.7881, 9.8343) knots 0 0 0 1 2 2 2
  line L153 (-2.7881, 9.8343) -> (-2.7881, 8.8084)
  line L154 (-2.7881, 8.8084) -> (-3.0409, 8.8084)
  line L155 (-3.0409, 8.8084) -> (-3.0409, 8.9672)
  line L156 (-3.0409, 9.1779) -> (-3.0409, 9.5944)
  spline S171 degree 2 poles (-3.0409, 9.5944) (-3.1317, 9.5863) (-3.4056, 9.5588) (-3.4915, 9.5329) knots 0 0 0 1 2 2 2
  spline S172 degree 2 poles (-3.4915, 9.5329) (-3.5919, 9.5021) (-3.7232, 9.374) (-3.7232, 9.2606) knots 0 0 0 1 2 2 2
  spline S173 degree 2 poles (-3.7232, 9.2606) (-3.7232, 9.1309) (-3.5774, 8.9996) (-3.438, 8.9996) knots 0 0 0 1 2 2 2
  spline S174 degree 2 poles (-3.438, 8.9996) (-3.3197, 8.9996) (-3.1252, 9.1017) (-3.0409, 9.1779) knots 0 0 0 1 2 2 2
  line L157 (-0.4201, 8.8084) -> (-0.673, 8.8084)
  line L158 (-0.673, 8.8084) -> (-0.673, 8.9607)
  spline S175 degree 2 poles (-0.673, 8.9607) (-0.7313, 8.9121) (-0.8172, 8.8473) (-0.8756, 8.8197) knots 0 0 0 1 2 2 2
  spline S176 degree 2 poles (-0.8756, 8.8197) (-0.9291, 8.7938) (-1.0441, 8.7662) (-1.1203, 8.7662) knots 0 0 0 1 2 2 2
  spline S177 degree 2 poles (-1.1203, 8.7662) (-1.2435, 8.7662) (-1.4509, 8.8684) (-1.5239, 8.9672) knots 0 0 0 1 2 2 2
  spline S178 degree 2 poles (-1.5239, 8.9672) (-1.5968, 9.0661) (-1.6778, 9.3578) (-1.6778, 9.5474) knots 0 0 0 1 2 2 2
  spline S179 degree 2 poles (-1.6778, 9.5474) (-1.6778, 9.7452) (-1.5757, 10.0337) (-1.4866, 10.1423) knots 0 0 0 1 2 2 2
  spline S180 degree 2 poles (-1.4866, 10.1423) (-1.4039, 10.2395) (-1.1722, 10.3513) (-1.0441, 10.3513) knots 0 0 0 1 2 2 2
  spline S181 degree 2 poles (-1.0441, 10.3513) (-0.9323, 10.3513) (-0.7654, 10.3011) (-0.673, 10.2492) knots 0 0 0 1 2 2 2
  line L159 (-0.673, 10.2492) -> (-0.673, 10.8975)
  line L160 (-0.673, 10.8975) -> (-0.4201, 10.8975)
  line L161 (-0.4201, 10.8975) -> (-0.4201, 8.8084)
  line L162 (-0.673, 9.1731) -> (-0.673, 10.0402)
  spline S182 degree 2 poles (-0.673, 10.0402) (-0.767, 10.0855) (-0.9161, 10.1196) (-1.002, 10.1196) knots 0 0 0 1 2 2 2
  spline S183 degree 2 poles (-1.002, 10.1196) (-1.1965, 10.1196) (-1.4169, 9.8278) (-1.4169, 9.5523) knots 0 0 0 1 2 2 2
  spline S184 degree 2 poles (-1.4169, 9.5523) (-1.4169, 9.2865) (-1.2483, 9.0061) (-1.062, 9.0061) knots 0 0 0 1 2 2 2
  spline S185 degree 2 poles (-1.062, 9.0061) (-0.9631, 9.0061) (-0.7621, 9.0969) (-0.673, 9.1731) knots 0 0 0 1 2 2 2
  spline S186 degree 2 poles (0.5977, 8.7743) (0.2379, 8.7743) (-0.1576, 9.1779) (-0.1576, 9.5507) knots 0 0 0 1 2 2 2
  spline S187 degree 2 poles (-0.1576, 9.5507) (-0.1576, 9.917) (0.2265, 10.3513) (0.5361, 10.3513) knots 0 0 0 1 2 2 2
  spline S188 degree 2 poles (0.5361, 10.3513) (0.6755, 10.3513) (0.891, 10.2703) (0.9705, 10.1844) knots 0 0 0 1 2 2 2
  spline S189 degree 2 poles (0.9705, 10.1844) (1.0515, 10.0985) (1.1374, 9.8505) (1.1374, 9.6706) knots 0 0 0 1 2 2 2
  line L163 (1.1374, 9.6706) -> (1.1374, 9.5329)
  line L164 (1.1374, 9.5329) -> (0.0985, 9.5329)
  spline S190 degree 2 poles (0.0985, 9.5329) (0.0985, 9.2719) (0.3611, 8.9948) (0.5944, 8.9948) knots 0 0 0 1 2 2 2
  spline S191 degree 2 poles (0.5944, 8.9948) (0.6771, 8.9948) (0.8376, 9.032) (0.9024, 9.0612) knots 0 0 0 1 2 2 2
  spline S192 degree 2 poles (0.9024, 9.0612) (0.9705, 9.0936) (1.0645, 9.1504) (1.0953, 9.1763) knots 0 0 0 1 2 2 2
  line L165 (1.0953, 9.1763) -> (1.1098, 9.1763)
  line L166 (1.1098, 9.1763) -> (1.1098, 8.9008)
  spline S193 degree 2 poles (1.1098, 8.9008) (1.0661, 8.8829) (0.9332, 8.8311) (0.8813, 8.8165) knots 0 0 0 1 2 2 2
  spline S194 degree 2 poles (0.8813, 8.8165) (0.8084, 8.7954) (0.6884, 8.7743) (0.5977, 8.7743) knots 0 0 0 1 2 2 2
  spline S195 degree 2 poles (0.891, 9.7257) (0.8878, 9.8278) (0.8457, 9.9769) (0.8051, 10.0272) knots 0 0 0 1 2 2 2
  spline S196 degree 2 poles (0.8051, 10.0272) (0.7614, 10.0839) (0.6236, 10.1439) (0.5215, 10.1439) knots 0 0 0 1 2 2 2
  spline S197 degree 2 poles (0.5215, 10.1439) (0.421, 10.1439) (0.28, 10.0839) (0.2217, 10.0256) knots 0 0 0 1 2 2 2
  spline S198 degree 2 poles (0.2217, 10.0256) (0.1649, 9.9656) (0.1066, 9.8214) (0.0985, 9.7257) knots 0 0 0 1 2 2 2
  line L167 (0.0985, 9.7257) -> (0.891, 9.7257)
  line L168 (1.6512, 8.8084) -> (1.3983, 8.8084)
  line L169 (1.3983, 8.8084) -> (1.3983, 10.8975)
  line L170 (1.3983, 10.8975) -> (1.6512, 10.8975)
  line L171 (1.6512, 10.8975) -> (1.6512, 8.8084)
  line L172 (2.28, 8.8084) -> (2.0272, 8.8084)
  line L173 (2.0272, 8.8084) -> (2.0272, 10.8975)
  line L174 (2.0272, 10.8975) -> (2.28, 10.8975)
  line L175 (2.28, 10.8975) -> (2.28, 8.8084)
  spline S199 degree 2 poles (3.3027, 8.7743) (2.9429, 8.7743) (2.5474, 9.1779) (2.5474, 9.5507) knots 0 0 0 1 2 2 2
  spline S200 degree 2 poles (2.5474, 9.5507) (2.5474, 9.917) (2.9316, 10.3513) (3.2411, 10.3513) knots 0 0 0 1 2 2 2
  spline S201 degree 2 poles (3.2411, 10.3513) (3.3805, 10.3513) (3.5961, 10.2703) (3.6755, 10.1844) knots 0 0 0 1 2 2 2
  spline S202 degree 2 poles (3.6755, 10.1844) (3.7565, 10.0985) (3.8424, 9.8505) (3.8424, 9.6706) knots 0 0 0 1 2 2 2
  line L176 (3.8424, 9.6706) -> (3.8424, 9.5329)
  line L177 (3.8424, 9.5329) -> (2.8035, 9.5329)
  spline S203 degree 2 poles (2.8035, 9.5329) (2.8035, 9.2719) (3.0661, 8.9948) (3.2995, 8.9948) knots 0 0 0 1 2 2 2
  spline S204 degree 2 poles (3.2995, 8.9948) (3.3821, 8.9948) (3.5426, 9.032) (3.6074, 9.0612) knots 0 0 0 1 2 2 2
  spline S205 degree 2 poles (3.6074, 9.0612) (3.6755, 9.0936) (3.7695, 9.1504) (3.8003, 9.1763) knots 0 0 0 1 2 2 2
  line L178 (3.8003, 9.1763) -> (3.8149, 9.1763)
  line L179 (3.8149, 9.1763) -> (3.8149, 8.9008)
  spline S206 degree 2 poles (3.8149, 8.9008) (3.7711, 8.8829) (3.6382, 8.8311) (3.5863, 8.8165) knots 0 0 0 1 2 2 2
  spline S207 degree 2 poles (3.5863, 8.8165) (3.5134, 8.7954) (3.3935, 8.7743) (3.3027, 8.7743) knots 0 0 0 1 2 2 2
  spline S208 degree 2 poles (3.5961, 9.7257) (3.5928, 9.8278) (3.5507, 9.9769) (3.5102, 10.0272) knots 0 0 0 1 2 2 2
  spline S209 degree 2 poles (3.5102, 10.0272) (3.4664, 10.0839) (3.3286, 10.1439) (3.2265, 10.1439) knots 0 0 0 1 2 2 2
  spline S210 degree 2 poles (3.2265, 10.1439) (3.126, 10.1439) (2.985, 10.0839) (2.9267, 10.0256) knots 0 0 0 1 2 2 2
  spline S211 degree 2 poles (2.9267, 10.0256) (2.87, 9.9656) (2.8116, 9.8214) (2.8035, 9.7257) knots 0 0 0 1 2 2 2
  line L180 (2.8035, 9.7257) -> (3.5961, 9.7257)
  line L181 (6.1358, 10.3092) -> (5.5701, 8.8084)
  line L182 (5.5701, 8.8084) -> (5.3432, 8.8084)
  line L183 (5.3432, 8.8084) -> (4.7825, 10.3092)
  line L184 (4.7825, 10.3092) -> (5.0564, 10.3092)
  line L185 (5.0564, 10.3092) -> (5.4664, 9.1536)
  line L186 (5.4664, 9.1536) -> (5.8732, 10.3092)
  line L187 (5.8732, 10.3092) -> (6.1358, 10.3092)
  line L188 (6.5847, 8.8084) -> (6.3319, 8.8084)
  line L189 (6.3319, 8.8084) -> (6.3319, 10.3092)
  line L190 (6.3319, 10.3092) -> (6.5847, 10.3092)
  line L191 (6.5847, 10.3092) -> (6.5847, 8.8084)
  line L192 (6.6025, 10.5588) -> (6.3157, 10.5588)
  line L193 (6.3157, 10.5588) -> (6.3157, 10.8214)
  line L194 (6.3157, 10.8214) -> (6.6025, 10.8214)
  line L195 (6.6025, 10.8214) -> (6.6025, 10.5588)
  spline S212 degree 2 poles (8.2136, 9.5831) (8.2136, 9.2152) (7.857, 8.7662) (7.588, 8.7662) knots 0 0 0 1 2 2 2
  spline S213 degree 2 poles (7.588, 8.7662) (7.4664, 8.7662) (7.293, 8.8262) (7.2087, 8.8781) knots 0 0 0 1 2 2 2
  line L196 (7.2087, 8.8781) -> (7.1925, 8.8084)
  line L197 (7.1925, 8.8084) -> (6.9559, 8.8084)
  line L198 (6.9559, 8.8084) -> (6.9559, 10.8975)
  line L199 (6.9559, 10.8975) -> (7.2087, 10.8975)
  line L200 (7.2087, 10.8975) -> (7.2087, 10.152)
  spline S214 degree 2 poles (7.2087, 10.152) (7.3043, 10.2379) (7.5264, 10.3513) (7.6674, 10.3513) knots 0 0 0 1 2 2 2
  spline S215 degree 2 poles (7.6674, 10.3513) (7.9218, 10.3513) (8.2136, 9.9445) (8.2136, 9.5831) knots 0 0 0 1 2 2 2
  spline S216 degree 2 poles (7.9526, 9.5637) (7.9526, 9.8327) (7.7889, 10.1115) (7.6074, 10.1115) knots 0 0 0 1 2 2 2
  spline S217 degree 2 poles (7.6074, 10.1115) (7.5053, 10.1115) (7.2946, 10.0142) (7.2087, 9.9397) knots 0 0 0 1 2 2 2
  line L201 (7.2087, 9.9397) -> (7.2087, 9.079)
  spline S218 degree 2 poles (7.2087, 9.079) (7.3043, 9.032) (7.4518, 8.9931) (7.5393, 8.9931) knots 0 0 0 1 2 2 2
  spline S219 degree 2 poles (7.5393, 8.9931) (7.7322, 8.9931) (7.9526, 9.2671) (7.9526, 9.5637) knots 0 0 0 1 2 2 2
  line L202 (9.2719, 10.0385) -> (9.2589, 10.0385)
  spline S220 degree 2 poles (9.2589, 10.0385) (9.2298, 10.0466) (9.1666, 10.0499) (9.1228, 10.0499) knots 0 0 0 1 2 2 2
  spline S221 degree 2 poles (9.1228, 10.0499) (9.0207, 10.0499) (8.8197, 9.9607) (8.729, 9.8732) knots 0 0 0 1 2 2 2
  line L203 (8.729, 9.8732) -> (8.729, 8.8084)
  line L204 (8.729, 8.8084) -> (8.4761, 8.8084)
  line L205 (8.4761, 8.8084) -> (8.4761, 10.3092)
  line L206 (8.4761, 10.3092) -> (8.729, 10.3092)
  line L207 (8.729, 10.3092) -> (8.729, 10.0855)
  spline S222 degree 2 poles (8.729, 10.0855) (8.8667, 10.2087) (9.0726, 10.3092) (9.1698, 10.3092) knots 0 0 0 1 2 2 2
  spline S223 degree 2 poles (9.1698, 10.3092) (9.2087, 10.3092) (9.2476, 10.306) (9.2719, 10.3011) knots 0 0 0 1 2 2 2
  line L208 (9.2719, 10.3011) -> (9.2719, 10.0385)
  spline S224 degree 2 poles (10.3043, 8.9672) (10.2735, 8.9445) (10.1698, 8.8635) (10.1212, 8.8392) knots 0 0 0 1 2 2 2
  spline S225 degree 2 poles (10.1212, 8.8392) (10.0547, 8.8035) (9.9299, 8.7662) (9.8165, 8.7662) knots 0 0 0 1 2 2 2
  spline S226 degree 2 poles (9.8165, 8.7662) (9.7241, 8.7662) (9.5572, 8.8359) (9.494, 8.8991) knots 0 0 0 1 2 2 2
  spline S227 degree 2 poles (9.494, 8.8991) (9.434, 8.9607) (9.3611, 9.1423) (9.3611, 9.2427) knots 0 0 0 1 2 2 2
  spline S228 degree 2 poles (9.3611, 9.2427) (9.3611, 9.3983) (9.4923, 9.6188) (9.635, 9.682) knots 0 0 0 1 2 2 2
  spline S229 degree 2 poles (9.635, 9.682) (9.7614, 9.7403) (10.105, 9.7841) (10.3043, 9.7954) knots 0 0 0 1 2 2 2
  line L209 (10.3043, 9.7954) -> (10.3043, 9.844)
  spline S230 degree 2 poles (10.3043, 9.844) (10.3043, 9.9316) (10.2508, 10.0402) (10.2022, 10.0709) knots 0 0 0 1 2 2 2
  spline S231 degree 2 poles (10.2022, 10.0709) (10.1536, 10.1017) (10.0142, 10.1212) (9.9397, 10.1212) knots 0 0 0 1 2 2 2
  spline S232 degree 2 poles (9.9397, 10.1212) (9.8521, 10.1212) (9.6155, 10.0693) (9.4972, 10.0191) knots 0 0 0 1 2 2 2
  line L210 (9.4972, 10.0191) -> (9.4826, 10.0191)
  line L211 (9.4826, 10.0191) -> (9.4826, 10.2768)
  spline S233 degree 2 poles (9.4826, 10.2768) (9.5523, 10.2962) (9.8132, 10.3449) (9.9413, 10.3449) knots 0 0 0 1 2 2 2
  spline S234 degree 2 poles (9.9413, 10.3449) (10.0969, 10.3449) (10.3092, 10.2962) (10.3935, 10.233) knots 0 0 0 1 2 2 2
  spline S235 degree 2 poles (10.3935, 10.233) (10.4761, 10.1714) (10.5572, 9.9753) (10.5572, 9.8343) knots 0 0 0 1 2 2 2
  line L212 (10.5572, 9.8343) -> (10.5572, 8.8084)
  line L213 (10.5572, 8.8084) -> (10.3043, 8.8084)
  line L214 (10.3043, 8.8084) -> (10.3043, 8.9672)
  line L215 (10.3043, 9.1779) -> (10.3043, 9.5944)
  spline S236 degree 2 poles (10.3043, 9.5944) (10.2136, 9.5863) (9.9397, 9.5588) (9.8538, 9.5329) knots 0 0 0 1 2 2 2
  spline S237 degree 2 poles (9.8538, 9.5329) (9.7533, 9.5021) (9.622, 9.374) (9.622, 9.2606) knots 0 0 0 1 2 2 2
  spline S238 degree 2 poles (9.622, 9.2606) (9.622, 9.1309) (9.7679, 8.9996) (9.9072, 8.9996) knots 0 0 0 1 2 2 2
  spline S239 degree 2 poles (9.9072, 8.9996) (10.0256, 8.9996) (10.2201, 9.1017) (10.3043, 9.1779) knots 0 0 0 1 2 2 2
  line L216 (11.8975, 8.8084) -> (10.7954, 8.8084)
  line L217 (10.7954, 8.8084) -> (10.7954, 8.9964)
  line L218 (10.7954, 8.9964) -> (11.5799, 10.1017)
  line L219 (11.5799, 10.1017) -> (10.8278, 10.1017)
  line L220 (10.8278, 10.1017) -> (10.8278, 10.3092)
  line L221 (10.8278, 10.3092) -> (11.8829, 10.3092)
  line L222 (11.8829, 10.3092) -> (11.8829, 10.1293)
  line L223 (11.8829, 10.1293) -> (11.0953, 9.0207)
  line L224 (11.0953, 9.0207) -> (11.8975, 9.0207)
  line L225 (11.8975, 9.0207) -> (11.8975, 8.8084)
  line L226 (12.3919, 8.8084) -> (12.139, 8.8084)
  line L227 (12.139, 8.8084) -> (12.139, 10.3092)
  line L228 (12.139, 10.3092) -> (12.3919, 10.3092)
  line L229 (12.3919, 10.3092) -> (12.3919, 8.8084)
  line L230 (12.4097, 10.5588) -> (12.1228, 10.5588)
  line L231 (12.1228, 10.5588) -> (12.1228, 10.8214)
  line L232 (12.1228, 10.8214) -> (12.4097, 10.8214)
  line L233 (12.4097, 10.8214) -> (12.4097, 10.5588)
  spline S240 degree 2 poles (13.9964, 9.5588) (13.9964, 9.1795) (13.6317, 8.7662) (13.327, 8.7662) knots 0 0 0 1 2 2 2
  spline S241 degree 2 poles (13.327, 8.7662) (13.0142, 8.7662) (12.656, 9.1925) (12.656, 9.5588) knots 0 0 0 1 2 2 2
  spline S242 degree 2 poles (12.656, 9.5588) (12.656, 9.9348) (13.0256, 10.3513) (13.327, 10.3513) knots 0 0 0 1 2 2 2
  spline S243 degree 2 poles (13.327, 10.3513) (13.6317, 10.3513) (13.9964, 9.9364) (13.9964, 9.5588) knots 0 0 0 1 2 2 2
  spline S244 degree 2 poles (13.7354, 9.5588) (13.7354, 9.8505) (13.5231, 10.1342) (13.327, 10.1342) knots 0 0 0 1 2 2 2
  spline S245 degree 2 poles (13.327, 10.1342) (13.1309, 10.1342) (12.917, 9.8505) (12.917, 9.5588) knots 0 0 0 1 2 2 2
  spline S246 degree 2 poles (12.917, 9.5588) (12.917, 9.2752) (13.1309, 8.9834) (13.327, 8.9834) knots 0 0 0 1 2 2 2
  spline S247 degree 2 poles (13.327, 8.9834) (13.5215, 8.9834) (13.7354, 9.2703) (13.7354, 9.5588) knots 0 0 0 1 2 2 2
  line L234 (15.434, 8.8084) -> (15.1812, 8.8084)
  line L235 (15.1812, 8.8084) -> (15.1812, 9.6641)
  spline S248 degree 2 poles (15.1812, 9.6641) (15.1812, 9.7679) (15.1617, 9.9461) (15.1325, 9.9996) knots 0 0 0 1 2 2 2
  spline S249 degree 2 poles (15.1325, 9.9996) (15.1017, 10.0564) (14.9915, 10.1115) (14.8975, 10.1115) knots 0 0 0 1 2 2 2
  spline S250 degree 2 poles (14.8975, 10.1115) (14.8035, 10.1115) (14.6042, 10.011) (14.5085, 9.9299) knots 0 0 0 1 2 2 2
  line L236 (14.5085, 9.9299) -> (14.5085, 8.8084)
  line L237 (14.5085, 8.8084) -> (14.2557, 8.8084)
  line L238 (14.2557, 8.8084) -> (14.2557, 10.3092)
  line L239 (14.2557, 10.3092) -> (14.5085, 10.3092)
  line L240 (14.5085, 10.3092) -> (14.5085, 10.1423)
  spline S251 degree 2 poles (14.5085, 10.1423) (14.622, 10.2444) (14.8408, 10.3513) (14.964, 10.3513) knots 0 0 0 1 2 2 2
  spline S252 degree 2 poles (14.964, 10.3513) (15.1844, 10.3513) (15.434, 10.0596) (15.434, 9.7825) knots 0 0 0 1 2 2 2
  line L241 (15.434, 9.7825) -> (15.434, 8.8084)
  line L242 (16.0466, 8.8084) -> (15.7938, 8.8084)
  line L243 (15.7938, 8.8084) -> (15.7938, 10.3092)
  line L244 (15.7938, 10.3092) -> (16.0466, 10.3092)
  line L245 (16.0466, 10.3092) -> (16.0466, 8.8084)
  line L246 (16.0645, 10.5588) -> (15.7776, 10.5588)
  line L247 (15.7776, 10.5588) -> (15.7776, 10.8214)
  line L248 (15.7776, 10.8214) -> (16.0645, 10.8214)
  line L249 (16.0645, 10.8214) -> (16.0645, 10.5588)
  line L250 (18.4729, 8.8084) -> (17.2395, 8.8084)
  line L251 (17.2395, 8.8084) -> (17.2395, 9.092)
  spline S253 degree 2 poles (17.2395, 9.092) (17.3724, 9.2168) (17.609, 9.4486) (17.7225, 9.5734) knots 0 0 0 1 2 2 2
  spline S254 degree 2 poles (17.7225, 9.5734) (17.951, 9.8246) (18.1179, 10.1261) (18.1179, 10.2865) knots 0 0 0 1 2 2 2
  spline S255 degree 2 poles (18.1179, 10.2865) (18.1179, 10.3708) (18.0661, 10.4972) (18.0191, 10.5377) knots 0 0 0 1 2 2 2
  spline S256 degree 2 poles (18.0191, 10.5377) (17.9721, 10.5782) (17.8489, 10.6188) (17.7743, 10.6188) knots 0 0 0 1 2 2 2
  spline S257 degree 2 poles (17.7743, 10.6188) (17.703, 10.6188) (17.5572, 10.5831) (17.4907, 10.5555) knots 0 0 0 1 2 2 2
  spline S258 degree 2 poles (17.4907, 10.5555) (17.434, 10.5329) (17.3286, 10.468) (17.2962, 10.4453) knots 0 0 0 1 2 2 2
  line L252 (17.2962, 10.4453) -> (17.2816, 10.4453)
  line L253 (17.2816, 10.4453) -> (17.2816, 10.7306)
  spline S259 degree 2 poles (17.2816, 10.7306) (17.3643, 10.7711) (17.6609, 10.8505) (17.7938, 10.8505) knots 0 0 0 1 2 2 2
  spline S260 degree 2 poles (17.7938, 10.8505) (18.0742, 10.8505) (18.3902, 10.5539) (18.3902, 10.3011) knots 0 0 0 1 2 2 2
  spline S261 degree 2 poles (18.3902, 10.3011) (18.3902, 10.1828) (18.3351, 9.985) (18.2865, 9.9008) knots 0 0 0 1 2 2 2
  spline S262 degree 2 poles (18.2865, 9.9008) (18.2379, 9.8132) (18.0969, 9.6414) (18.0191, 9.5588) knots 0 0 0 1 2 2 2
  spline S263 degree 2 poles (18.0191, 9.5588) (17.8927, 9.421) (17.5831, 9.1261) (17.4907, 9.0402) knots 0 0 0 1 2 2 2
  line L254 (17.4907, 9.0402) -> (18.4729, 9.0402)
  line L255 (18.4729, 9.0402) -> (18.4729, 8.8084)
  spline S264 degree 2 poles (19.985, 9.8084) (19.985, 9.2703) (19.6722, 8.7662) (19.3465, 8.7662) knots 0 0 0 1 2 2 2
  spline S265 degree 2 poles (19.3465, 8.7662) (19.0158, 8.7662) (18.7063, 9.28) (18.7063, 9.8068) knots 0 0 0 1 2 2 2
  spline S266 degree 2 poles (18.7063, 9.8068) (18.7063, 10.3481) (19.0191, 10.8489) (19.3465, 10.8489) knots 0 0 0 1 2 2 2
  spline S267 degree 2 poles (19.3465, 10.8489) (19.6755, 10.8489) (19.985, 10.3303) (19.985, 9.8084) knots 0 0 0 1 2 2 2
  spline S268 degree 2 poles (19.6414, 9.199) (19.6803, 9.2978) (19.7128, 9.6026) (19.7128, 9.8084) knots 0 0 0 1 2 2 2
  spline S269 degree 2 poles (19.7128, 9.8084) (19.7128, 10.0142) (19.6803, 10.3173) (19.6398, 10.4194) knots 0 0 0 1 2 2 2
  spline S270 degree 2 poles (19.6398, 10.4194) (19.5993, 10.5215) (19.4583, 10.6269) (19.3465, 10.6269) knots 0 0 0 1 2 2 2
  spline S271 degree 2 poles (19.3465, 10.6269) (19.2346, 10.6269) (19.0904, 10.5215) (19.0483, 10.4162) knots 0 0 0 1 2 2 2
  spline S272 degree 2 poles (19.0483, 10.4162) (19.0077, 10.3141) (18.9786, 10.0029) (18.9786, 9.8068) knots 0 0 0 1 2 2 2
  spline S273 degree 2 poles (18.9786, 9.8068) (18.9786, 9.5961) (19.0045, 9.3141) (19.0466, 9.2038) knots 0 0 0 1 2 2 2
  spline S274 degree 2 poles (19.0466, 9.2038) (19.0855, 9.1001) (19.2298, 8.9883) (19.3465, 8.9883) knots 0 0 0 1 2 2 2
  spline S275 degree 2 poles (19.3465, 8.9883) (19.4567, 8.9883) (19.6009, 9.0936) (19.6414, 9.199) knots 0 0 0 1 2 2 2
  line L256 (21.374, 8.8084) -> (20.3983, 8.8084)
  line L257 (20.3983, 8.8084) -> (20.3983, 9.0126)
  line L258 (20.3983, 9.0126) -> (20.7614, 9.0126)
  line L259 (20.7614, 9.0126) -> (20.7614, 10.353)
  line L260 (20.7614, 10.353) -> (20.3983, 10.353)
  line L261 (20.3983, 10.353) -> (20.3983, 10.5361)
  spline S276 degree 2 poles (20.3983, 10.5361) (20.6042, 10.5361) (20.7987, 10.6528) (20.8116, 10.8149) knots 0 0 0 1 2 2 2
  line L262 (20.8116, 10.8149) -> (21.0191, 10.8149)
  line L263 (21.0191, 10.8149) -> (21.0191, 9.0126)
  line L264 (21.0191, 9.0126) -> (21.374, 9.0126)
  line L265 (21.374, 9.0126) -> (21.374, 8.8084)
  spline S277 degree 2 poles (21.6868, 10.1585) (21.6868, 10.3124) (21.7873, 10.5685) (21.8748, 10.6609) knots 0 0 0 1 2 2 2
  spline S278 degree 2 poles (21.8748, 10.6609) (21.9575, 10.75) (22.199, 10.8489) (22.3222, 10.8489) knots 0 0 0 1 2 2 2
  spline S279 degree 2 poles (22.3222, 10.8489) (22.4599, 10.8489) (22.6836, 10.7565) (22.7662, 10.669) knots 0 0 0 1 2 2 2
  spline S280 degree 2 poles (22.7662, 10.669) (22.87, 10.5588) (22.9834, 10.2022) (22.9834, 9.9283) knots 0 0 0 1 2 2 2
  spline S281 degree 2 poles (22.9834, 9.9283) (22.9834, 9.6803) (22.8716, 9.2363) (22.763, 9.0888) knots 0 0 0 1 2 2 2
  spline S282 degree 2 poles (22.763, 9.0888) (22.6479, 8.9332) (22.3238, 8.7695) (22.0872, 8.7695) knots 0 0 0 1 2 2 2
  spline S283 degree 2 poles (22.0872, 8.7695) (22.0337, 8.7695) (21.9121, 8.7808) (21.8602, 8.797) knots 0 0 0 1 2 2 2
  line L266 (21.8602, 8.797) -> (21.8602, 9.0547)
  line L267 (21.8602, 9.0547) -> (21.8732, 9.0547)
  spline S284 degree 2 poles (21.8732, 9.0547) (21.9072, 9.0353) (22.0499, 9.0013) (22.1228, 9.0013) knots 0 0 0 1 2 2 2
  spline S285 degree 2 poles (22.1228, 9.0013) (22.3854, 9.0013) (22.6852, 9.3481) (22.7063, 9.669) knots 0 0 0 1 2 2 2